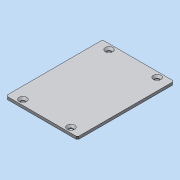
# Autodesk Inventor part: BC-10023
Saved by Autodesk Inventor 2016 (Build 200138000, 138)
## iProperties
Created: 2015-12-01
Part Number: BC-10023
Project: DIPOLO BC-3T- SIRIUS
Cost Center: 0.00.00.000
Material: Alumínio 7075
Document SubType Name: Modeling
Designer: reinaldo.basilio
Density: 2.81 g/cm^3
Appearance: Satin - Brushed Heavy
Description: Proteção dos blocos laterais.
Mass: 162.325 g
Surface Area: 311.637 cm^2
Volume: 57.7668 cm^3
RuleStatus: InUse
AfterMaterialChange0: file://_iMaterial
AfterAnyiPropertyChange0: file://_iMaterial
AfterDocNew0: file://_Naming_par
AfterDocNew1: file://_NameStart
AfterDocNew2: file://_NameStart1
AfterDocNew3: file://_Materiais
DocNumber: XXXXX-XXX-XXXX-00-001.ipt
Folder: .
Title: DIPOLO BC-3T- SIRIUS
Author: reinaldo.basilio
Subject: BC-10023
Autodesk Inventor part; units mm, degrees
ref_plane "YZ Plane" through (0, 0, 0) normal (1, 0, 0) x (0, 1, 0)
ref_plane "XZ Plane" through (0, 0, 0) normal (0, 1, 0) x (-1, 0, 0)
ref_plane "XY Plane" through (0, 0, 0) normal (0, 0, 1) x (1, 0, 0)
sketch "Sketch5" plane through (0, 0, 0) normal (0, 0, 1) x (1, 0, 0)
  line L0 (-70.25, 52) -> (70.25, 52)
  line L1 (70.25, 52) -> (70.25, -52)
  line L2 (70.25, -52) -> (-70.25, -52)
  line L3 (-70.25, -52) -> (-70.25, 52)
  point P0 (0, 0)
  point P1 (0, 52)
  point P2 (70.25, 0)
  dimension "d8" = 140.5
  dimension "d9" = 104
  constraints: 8 end point, 2 midpoint, 2 parallel, 1 horizontal, 1 horizontal alignment, 1 perpendicular, 1 vertical alignment
  measures "d8" distance of L0.start L0.end
  measures "d9" distance of L2.end L0.start
extrude "Extrusion5" add sketch "Sketch5" along normal blind 4
sketch "Sketch6" plane through (0, 0, 4) normal (0, 0, 1) x (1, 0, 0)
  circle A0 centre (-62.75, 35) radius 3
  circle A1 centre (-62.75, -35) radius 3
  circle A2 centre (62.75, 35) radius 3
  circle A3 centre (62.75, -35) radius 3
  line L0 (-70.25, 52) -> (-70.25, -52) projected
  line L1 (-70.25, -52) -> (70.25, -52) projected
  point P0 (0, 0)
  point P1 (0, 0)
  point P2 (0, -52)
  point P3 (-70.25, 0)
  dimension "d19" = 125.5
  dimension "d20" = 62.75
  dimension "d21" = 70
  dimension "d22" = 35
  dimension "d23" = 6
  constraints: 4 centre point, 3 equal radius, 3 horizontal alignment, 3 vertical alignment, 2 midpoint
  measures "d19" distance of A2.centre A0.centre
  measures "d20" horizontal distance of point (0, 0) A0.centre
  measures "d21" distance of A1.centre A0.centre
  measures "d22" vertical distance of point (0, 0) A1.centre
  measures "d23" diameter of A0
hole "Hole1" at (-62.75, 35, 4) at (62.75, 35, 4) at (62.75, -35, 4) at (-62.75, -35, 4) direction (0, 0, -1) diameter 5.5 end through all countersink diameter 11 countersink angle 90 clearance for "Countersunk Flat Head Screw DIN EN ISO 2009" size "M5" standard "DIN"
chamfer "Chamfer1" distance 2 angle 45 4 edges at (70.25, -52, 2) (70.25, 52, 2) (-70.25, 52, 2) (-70.25, -52, 2)
equation "\"d20\" = 0.5 * d19"
equation "\"d22\" = 0.5 * d21"
body "Solid5"
